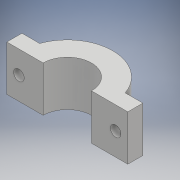
# Autodesk Inventor part: prism_holder_2
Saved by Autodesk Inventor 2018 (Build 220112000, 112)
## iProperties
Created: 2017-11-13
Part Number: prism_holder_2
Material: Generic
Document SubType Name: Modeling
Designer: Bardo91
Density: 1 g/cm^3
Appearance: Default
Author: Bardo91
Autodesk Inventor part; units mm, degrees
ref_plane "YZ Plane" through (0, 0, 0) normal (1, 0, 0) x (0, 1, 0)
ref_plane "XZ Plane" through (0, 0, 0) normal (0, 1, 0) x (-1, 0, 0)
ref_plane "XY Plane" through (0, 0, 0) normal (0, 0, 1) x (1, 0, 0)
sketch "Sketch1" plane through (0, 0, 0) normal (0, 0, 1) x (1, 0, 0)
  arc A0 (8, 0) -> (-8, 0) centre (0, 0) ccw
  arc A1 (15, 0) -> (-15, 0) centre (0, 0) ccw
  line L0 (-8, 0) -> (-15, 0)
  line L1 (-15, 0) -> (-20, 0)
  line L2 (-20, 0) -> (-20, 5)
  line L3 (-20, 5) -> (-14.1421, 5)
  line L4 (8, 0) -> (15, 0)
  line L5 (15, 0) -> (20, 0)
  line L6 (20, 0) -> (20, 5)
  line L7 (20, 5) -> (14.1421, 5)
  dimension "d0" = 16
  dimension "d1" = 30
  dimension "d2" = 5
  dimension "d3" = 5
  dimension "d4" = 5
  dimension "d5" = 5
  constraints: 16 end point, 6 point on circle, 6 point on line, 2 centre point, 2 coincident, 2 perpendicular, 1 horizontal
  measures "d0" diameter of A0
  measures "d1" diameter of A1
  measures "d2" distance of L0.end L1.end
  measures "d3" distance of L1.end L2.end
  measures "d4" distance of L4.end L5.end
  measures "d5" distance of L5.end L6.end
extrude "Extrusion1" add sketch "Sketch1" along normal blind 15
sketch "Sketch2" plane through (8, 0, 0) normal (0, -1, 0) x (1, 0, 0)
  line L0 (-28, 0) -> (-28, 15) projected
  line L1 (-28, 7.5) -> (-24, 7.5)
  line L2 (12, 0) -> (12, 15) projected
  line L3 (12, 7.5) -> (8, 7.5)
  circle A0 centre (-24, 7.5) radius 1.75
  circle A1 centre (8, 7.5) radius 1.75
  point P0 (-8, 0)
  dimension "d8" = 4
  dimension "d9" = 4
  dimension "d10" = 3.5
  dimension "d11" = 3.5
  constraints: 4 end point, 2 centre point, 2 coincident, 2 horizontal, 2 midpoint
  measures "d8" distance of L1.start L1.end
  measures "d9" distance of L3.start L3.end
  measures "d10" diameter of A0
  measures "d11" diameter of A1
extrude "Extrusion2" cut sketch "Sketch2" against normal through all
body "Solid1"
